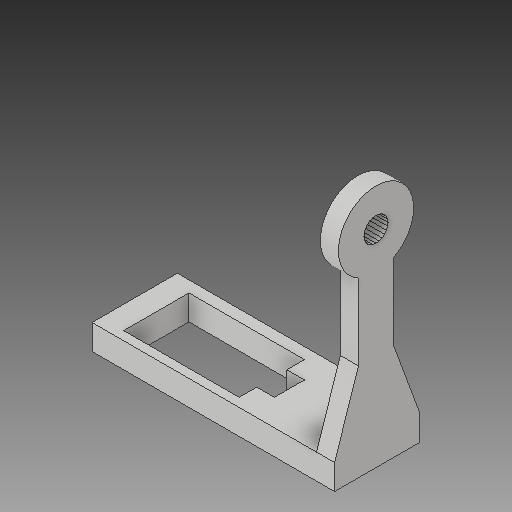
# Autodesk Inventor part: arm
Saved by Autodesk Inventor 2019 (Build 230136000, 136)
## iProperties
Created: 2020-04-01
Part Number: arm
Material: Generic
Document SubType Name: Modeling
Designer: Pulag
Density: 1 g/cm^3
Appearance: Default
Author: Pulag
Autodesk Inventor part; units mm, degrees
ref_plane "YZ Plane" through (0, 0, 0) normal (1, 0, 0) x (0, 1, 0)
ref_plane "XZ Plane" through (0, 0, 0) normal (0, 1, 0) x (-1, 0, 0)
ref_plane "XY Plane" through (0, 0, 0) normal (0, 0, 1) x (1, 0, 0)
sketch "Sketch1" plane through (0, 0, 0) normal (0, 0, 1) x (1, 0, 0)
  line L0 (-27.3, -5) -> (21, -5)
  line L1 (21, 0) -> (-27.3, 0)
  line L2 (-27.3, 0) -> (-27.3, -5)
  line L3 (17.4, 46.3236) -> (17.4, 0)
  line L4 (17.4, 0) -> (21, 0)
  line L5 (21, 41.8826) -> (21, 41.2832) projected
  line L6 (17.4, 46.3236) -> (21, 46.3236)
  line L7 (21, 46.3236) -> (21, 0)
  line L8 (21, 0) -> (17.4, 0)
  line L9 (17.4, 0) -> (17.4, 46.3236)
  line L10 (21, 0) -> (21, -5)
  point P0 (0, 0)
  point P1 (-27.3, 0)
  point P2 (17.4, 38.1655)
  constraints: 20 end point, 3 parallel, 2 horizontal, 2 point on line, 1 perpendicular, 1 vertical, 1 other
extrude "Extrusion1" add sketch "Sketch1" against normal blind 15
sketch "Sketch2" plane through (0, 0, 0) normal (0, 0, 1) x (1, 0, 0)
  line L0 (17.4, 0) -> (-27.3, 0) projected
  line L1 (-27.3, 0) -> (-27.3, -5) projected
  line L2 (21, -5) -> (21, 46.3236) projected
  line L3 (21, 46.3236) -> (17.4, 46.3236) projected
  line L4 (17.4, 46.3236) -> (17.4, 0) projected
  line L5 (-27.3, -5) -> (21, -5) projected
  point P0 (0, 0)
extrude "Extrusion2" add sketch "Sketch2" along normal blind 2
sketch "Sketch3" plane through (17.4, 0, -15) normal (-1, 0, 0) x (0, 0, 1)
  line L0 (10.8285, 34.887) -> (11.0682, 35.4658) projected
  line L1 (11.15, 36.087) -> (11.0682, 35.4658) projected
  line L2 (11.0682, 36.7082) -> (11.15, 36.087) projected
  line L3 (10.8285, 37.287) -> (11.0682, 36.7082) projected
  line L4 (10.4471, 37.7841) -> (10.8285, 37.287) projected
  line L5 (9.95, 38.1655) -> (10.4471, 37.7841) projected
  line L6 (9.3712, 38.4052) -> (9.95, 38.1655) projected
  line L7 (9.3712, 38.4052) -> (8.75, 38.487) projected
  line L8 (8.1288, 38.4052) -> (8.75, 38.487) projected
  line L9 (8.1288, 38.4052) -> (7.55, 38.1655) projected
  line L10 (7.55, 38.1655) -> (7.0529, 37.7841) projected
  line L11 (7.0529, 37.7841) -> (6.6715, 37.287) projected
  line L12 (6.6715, 37.287) -> (6.4318, 36.7082) projected
  line L13 (6.4318, 36.7082) -> (6.35, 36.087) projected
  line L14 (6.35, 36.087) -> (6.4318, 35.4658) projected
  line L15 (6.4318, 35.4658) -> (6.6715, 34.887) projected
  line L16 (6.6715, 34.887) -> (7.0529, 34.3899) projected
  line L17 (7.0529, 34.3899) -> (7.55, 34.0085) projected
  line L18 (8.1288, 33.7688) -> (7.55, 34.0085) projected
  line L19 (8.1288, 33.7688) -> (8.75, 33.687) projected
  line L20 (8.75, 33.687) -> (9.3712, 33.7688) projected
  line L21 (9.3712, 33.7688) -> (9.95, 34.0085) projected
  line L22 (9.95, 34.0085) -> (10.4471, 34.3899) projected
  line L23 (10.8285, 34.887) -> (10.4471, 34.3899) projected
  line L24 (8.75, 35.087) -> (9.0088, 35.1211) projected
  line L25 (8.4912, 35.1211) -> (8.75, 35.087) projected
  line L26 (8.25, 35.221) -> (8.4912, 35.1211) projected
  line L27 (8.0429, 35.3799) -> (8.25, 35.221) projected
  line L28 (7.884, 35.587) -> (8.0429, 35.3799) projected
  line L29 (7.7841, 35.8282) -> (7.884, 35.587) projected
  line L30 (7.75, 36.087) -> (7.7841, 35.8282) projected
  line L31 (7.7841, 36.3458) -> (7.75, 36.087) projected
  line L32 (7.884, 36.587) -> (7.7841, 36.3458) projected
  line L33 (8.0429, 36.7941) -> (7.884, 36.587) projected
  line L34 (8.25, 36.953) -> (8.0429, 36.7941) projected
  line L35 (8.4912, 37.0529) -> (8.25, 36.953) projected
  line L36 (8.75, 37.087) -> (8.4912, 37.0529) projected
  line L37 (8.75, 37.087) -> (9.0088, 37.0529) projected
  line L38 (9.0088, 37.0529) -> (9.25, 36.953) projected
  line L39 (9.25, 36.953) -> (9.4571, 36.7941) projected
  line L40 (9.4571, 36.7941) -> (9.616, 36.587) projected
  line L41 (9.616, 36.587) -> (9.7159, 36.3458) projected
  line L42 (9.7159, 36.3458) -> (9.75, 36.087) projected
  line L43 (9.75, 36.087) -> (9.7159, 35.8282) projected
  line L44 (9.7159, 35.8282) -> (9.616, 35.587) projected
  line L45 (9.616, 35.587) -> (9.4571, 35.3799) projected
  line L46 (9.4571, 35.3799) -> (9.25, 35.221) projected
  line L47 (9.25, 35.221) -> (9.0088, 35.1211) projected
  circle A0 centre (8.75, 36.087) radius 2.5
  arc A1 (12.25, 29.4537) -> (5.25, 29.4537) centre (8.75, 36.087) ccw
  line L48 (8.75, 36.087) -> (8.75, 28.587)
  line L49 (0, 0) -> (17, 0) projected
  line L50 (0, -5) -> (0, 0) projected
  line L51 (0, -5) -> (17, -5) projected
  line L52 (17, 0) -> (17, -5) projected
  line L53 (8.75, 28.587) -> (8.75, 0)
  line L54 (0, 0) -> (17, 0) projected
  line L55 (5.25, 14.2935) -> (5.25, 28.587)
  line L56 (12.25, 28.587) -> (12.25, 14.2935)
  line L57 (12.25, 0) -> (5.25, 0)
  line L58 (5.25, 0) -> (12.25, 28.587) construction
  line L59 (5.25, 28.587) -> (12.25, 0) construction
  line L60 (12.25, 28.587) -> (12.25, 29.4537)
  line L61 (5.25, 28.587) -> (5.25, 29.4537)
  line L62 (0, 46.3236) -> (17, 46.3236) projected
  line L63 (17, 46.3236) -> (0, 46.3236)
  line L64 (0, 46.3236) -> (0, 0)
  line L65 (0, 0) -> (17, 0)
  line L66 (17, 0) -> (17, 46.3236)
  line L67 (5.25, 14.2935) -> (0, 0)
  line L68 (12.25, 14.2935) -> (17, 0)
  point P0 (15, 0)
  point P1 (8.75, 14.2935)
  dimension "d6" = 5
  dimension "d7" = 15
  dimension "d8" = 7
  constraints: 30 end point, 5 parallel, 3 midpoint, 2 centre point, 2 coincident, 2 perpendicular, 2 point on circle, 2 vertical, 1 horizontal, 1 point on line
  measures "d6" diameter of A0
  measures "d7" diameter of A1
  measures "d8" distance of L55.end L56.start
extrude "Extrusion3" cut sketch "Sketch3" against normal up to surface (3.6 mm away) contours L25 L26 L27 L28 L29 L30 L31 L32 L33 L34 L35 L36 L37 L38 L39 L40 L41 L42 L43 L44 L45 L46 L47 L24 | L23 L22 L21 L20 L19 L18 L17 L16 L15 L14 L13 L12 L11 L10 L9 L8 L7 L6 L5 L4 L3 L2 L1 L0 | L64 L62 L66 L68 L56 L60 A1 L61 L55 L67
sketch "Sketch5" plane through (-27.3, -5, -15) normal (0, -1, 0) x (1, 0, 0)
  line L0 (4.8, 15) -> (4.8, 2.5) projected
  line L1 (27.3, 15) -> (4.8, 15) projected
  line L2 (27.3, 2.5) -> (27.3, 15) projected
  line L3 (27.3, 2.5) -> (4.8, 2.5) projected
  line L4 (4.8, 2.5) -> (27.3, 15)
  line L5 (27.55, 2.25) -> (4.55, 2.25)
  line L6 (4.55, 2.25) -> (4.55, 15.25)
  line L7 (4.55, 15.25) -> (27.55, 15.25)
  line L8 (27.55, 15.25) -> (27.55, 2.25)
  line L9 (27.55, 2.25) -> (4.55, 15.25) construction
  line L10 (4.55, 2.25) -> (27.55, 15.25) construction
  line L11 (27.55, 5.75) -> (31.05, 5.75)
  line L12 (31.05, 5.75) -> (31.05, 11.75)
  line L13 (31.05, 11.75) -> (27.55, 11.75)
  line L14 (24.05, 5.75) -> (31.05, 11.75) construction
  line L15 (31.05, 5.75) -> (24.05, 11.75) construction
  point P0 (16.05, 8.75)
  point P1 (27.55, 8.75)
  dimension "d11" = 23
  dimension "d12" = 13
  dimension "d13" = 7
  dimension "d14" = 6
  constraints: 24 end point, 6 midpoint, 3 parallel, 2 horizontal, 2 perpendicular, 2 point on line
  measures "d11" distance of L6.end L7.end
  measures "d12" distance of L5.end L6.end
  measures "d13" distance of L15.end L12.end
  measures "d14" distance of L12.end L11.end
extrude "Extrusion4" cut sketch "Sketch5" against normal up to surface (5 mm away) contours L1 L4 L0 | L4 L2 L3 | L5 L6 L7 L8 | L8 L13 L12 L11
body "Solid1"
